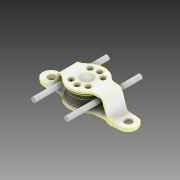
# Autodesk Inventor part: Harken 22mm Cheek
Saved by Autodesk Inventor 2022 (Build 260153000, 153)
## iProperties
Created: 2013-05-03
Part Number: Harken 22mm Cheek
Material: Aluminum 6061
Description: SolidWorks IGES file using analytic representation for surfaces
Document SubType Name: Modeling
Designer: Nemo
Mass: 21 g
Density: 2.7 g/cm^3
Appearance: Default
Title: \\ntserver\ENGINEER\catalog eng files\NEW\233.IGS
Author: mallory.siguenza
Sending System: SolidWorks 2011
Preprocessor: SolidWorks 2011
Minimum Resolution: 0.0
Sending System Product ID: 233.SLDPRT
Receiving System Product ID: 233.SLDPRT
Sent Units: Centimeter
Translation Standard: IGES 5.3
Model Creation Time: 2013-05-03
Density: 1.06097 g/cm^3
Surface Area: 10.2912 cm^2
Volume: 0.79173 cm^3
Autodesk Inventor part; units mm, degrees
ref_plane "YZ Plane" through (0, 0, 0) normal (1, 0, 0) x (0, 1, 0)
ref_plane "XZ Plane" through (0, 0, 0) normal (0, 1, 0) x (-1, 0, 0)
ref_plane "XY Plane" through (0, 0, 0) normal (0, 0, 1) x (1, 0, 0)
surface "Composite1"
sketch "Sketch2" plane through (0, 0, 0) normal (0, 0, 1) x (1, 0, 0)
  line L0 (39.5181, -1.4448) -> (22.0101, -1.4448) projected
  circle A0 centre (20.4226, -1.4448) radius 1.5875
  line L1 (23.7903, -1.4448) -> (41.2982, -1.4448) projected
  circle A1 centre (42.8857, -1.4448) radius 1.5875
  line L2 (20.4226, -1.4448) -> (42.8857, -1.4448) construction
  point P0 (0, 0)
  dimension "d1" = 3.175
  constraints: 2 end point, 2 horizontal alignment, 1 horizontal, 1 point on line, 4 other
extrude "Extrusion1" add sketch "Sketch2" against normal mid plane 50
body "Solid1"
body "Srf1"
